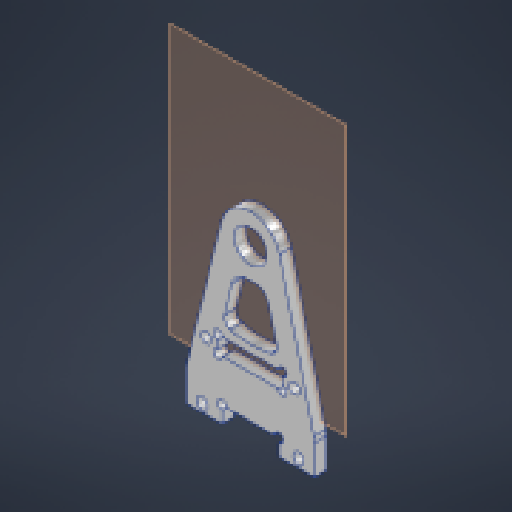
# Autodesk Inventor part: Roll_Fixation_Frame_2t1
Saved by Autodesk Inventor 2024 (Build 280153000, 153)
## iProperties
Created: 2024-01-23
Part Number: Roll_Fixation_Frame_2t1
Material: 알루미늄 6061
Document SubType Name: Modeling
Designer: ASUS
Density: 2.7 g/cm^3
Appearance: 알루미늄 - 평지
Author: ASUS
Autodesk Inventor part; units mm, degrees
(part 1 of 3)
ref_plane "YZ Plane" through (0, 0, 0) normal (1, 0, 0) x (0, 1, 0)
ref_plane "XZ Plane" through (0, 0, 0) normal (0, 1, 0) x (-1, 0, 0)
ref_plane "XY Plane" through (0, 0, 0) normal (0, 0, 1) x (1, 0, 0)
ref_plane "작업 평면1" through (0, 0, 0) normal (0, 0, 1) x (1, 0, 0)
sketch "스케치1" plane through (0, 0, 0) normal (0, 0, 1) x (1, 0, 0)
  circle A0 centre (0.1, -20) radius 6 projected
  circle A1 centre (0.1, -20) radius 4 projected
  line L0 (-13.4121, -48.1) -> (13.4121, -48.1) projected
  line L1 (0.1, -20) -> (0.1, -60)
  line L2 (0.1, -60) -> (-15.9, -60)
  line L3 (-15.9, -60) -> (-5.7269, -18.5692)
  line L4 (0.1, -60) -> (16.1, -60)
  line L5 (16.1, -60) -> (5.9269, -18.5692)
  line L6 (0.1, -48.1) -> (0.1, -60)
  line L7 (7.6, -52.05) -> (-7.4, -52.05)
  line L8 (-7.4, -52.05) -> (-7.4, -56.05)
  line L9 (-7.4, -56.05) -> (7.6, -56.05)
  line L10 (7.6, -56.05) -> (7.6, -52.05)
  line L11 (7.6, -52.05) -> (-7.4, -56.05) construction
  line L12 (-7.4, -52.05) -> (7.6, -56.05) construction
  line L13 (-7.4, -54.05) -> (-10.4, -54.05)
  line L14 (7.6, -54.05) -> (10.6, -54.05)
  circle A2 centre (10.6, -54.05) radius 1.35
  circle A3 centre (-10.4, -54.05) radius 1.35
  line L15 (7.6, -56.05) -> (7.6, -52.05) construction
  line L16 (-34.247, -53.3276) -> (-34.247, -49.3276)
  line L17 (-37.747, -49.3276) -> (-37.747, -53.3276)
  arc A4 (-37.747, -53.3276) -> (-34.247, -53.3276) centre (-35.997, -53.3276) ccw
  arc A5 (-34.247, -49.3276) -> (-37.747, -49.3276) centre (-35.997, -49.3276) ccw
  line L18 (4.1, -52.05) -> (4.1, -56.05)
  line L19 (7.6, -56.05) -> (7.6, -52.05)
  arc A6 (7.6, -52.05) -> (4.1, -52.05) centre (5.85, -52.05) ccw
  arc A7 (4.1, -56.05) -> (7.6, -56.05) centre (5.85, -56.05) ccw
  line L20 (-7.4, -52.05) -> (-7.4, -56.05)
  line L21 (-3.9, -56.05) -> (-3.9, -52.05)
  arc A8 (-3.9, -52.05) -> (-7.4, -52.05) centre (-5.65, -52.05) ccw
  arc A9 (-7.4, -56.05) -> (-3.9, -56.05) centre (-5.65, -56.05) ccw
  line L22 (-10.4, -54.05) -> (-22.3103, -54.05)
  line L23 (-22.3103, -54.05) -> (17.7315, -54.05)
  line L24 (14.639, -54.05) -> (-14.439, -54.05)
  line L25 (-14.439, -54.05) -> (-14.439, -60)
  line L26 (-14.439, -60) -> (14.639, -60)
  line L27 (14.639, -60) -> (14.639, -54.05)
  point P0 (0, 0)
  point P1 (0.1, -54.05)
  point P2 (-32.997, -51.3276)
  point P3 (-2.65, -54.05)
  point P4 (7.6, -56.05)
  point P5 (4.1, -56.05)
  point P6 (-7.4, -52.05)
  point P7 (5.9269, -18.5692)
  dimension "d0" = 40
  dimension "d1" = 16
  dimension "d2" = 15
  dimension "d3" = 4
  dimension "d4" = 3
  dimension "d5" = 3
  dimension "d7" = 2.7
  constraints: 56 end point, 12 point on circle, 12 tangent, 8 centre point, 7 parallel, 7 point on line, 6 midpoint, 5 horizontal, 4 perpendicular, 2 coincident, 2 symmetric about line, 1 vertical, 3 other
  measures "d0" distance of L1.start L1.end
  measures "d1" distance of L1.end L2.end
  measures "d2" distance of L9.end L8.end
  measures "d3" distance of L8.end L7.end
  measures "d4" distance of L13.start L13.end
  measures "d5" distance of L14.start L14.end
  measures "d7" diameter of A3
extrude "돌출1" add sketch "스케치1" along normal blind 3 contours A0 | A0 L5 L0 L1 | L1 L0 L3 A0 | L5 L23 A2 L14 L10 A6 L7 L1 L0 | L1 L7 A8 L8 L13 A3 L22 L3 L0 | L27 L4 L1 L9 A7 L10 L14 A2 L23 | L22 A3 L13 L8 A9 L9 L1 L2 L25
fillet "모깎기1" radius 4 2 edges at (14.639, -60, 1.5) (-14.439, -60, 1.5)
sketch "스케치2" plane through (0, 0, 3) normal (0, 0, 1) x (1, 0, 0)
  arc A0 (-14.439, -56) -> (-10.439, -60) centre (-10.439, -56) ccw projected
  line L0 (-10.439, -60) -> (10.639, -60) projected
  arc A1 (10.639, -60) -> (14.639, -56) centre (10.639, -56) ccw projected
  line L1 (14.639, -56) -> (14.639, -54.05) projected
  line L2 (14.639, -54.05) -> (5.9269, -18.5692) projected
  arc A2 (5.9269, -18.5692) -> (-5.7269, -18.5692) centre (0.1, -20) ccw projected
  line L3 (-5.7269, -18.5692) -> (-14.439, -54.05) projected
  line L4 (-14.439, -54.05) -> (-14.439, -56) projected
  line L5 (7.6, -52.05) -> (7.6, -56.05) projected
  arc A3 (4.1, -56.05) -> (7.6, -56.05) centre (5.85, -56.05) ccw projected
  line L6 (4.1, -56.05) -> (-3.9, -56.05) projected
  arc A4 (-7.4, -56.05) -> (-3.9, -56.05) centre (-5.65, -56.05) ccw projected
  line L7 (-7.4, -56.05) -> (-7.4, -52.05) projected
  arc A5 (-3.9, -52.05) -> (-7.4, -52.05) centre (-5.65, -52.05) ccw projected
  line L8 (-3.9, -52.05) -> (4.1, -52.05) projected
  arc A6 (7.6, -52.05) -> (4.1, -52.05) centre (5.85, -52.05) ccw projected
  circle A7 centre (10.6, -54.05) radius 1.35 projected
  circle A8 centre (0.1, -20) radius 4 projected
  circle A9 centre (-10.4, -54.05) radius 1.35 projected
  line L9 (-10.439, -54.5339) -> (-1.8423, -19.5231)
  arc A10 (2.0423, -19.5231) -> (-1.8423, -19.5231) centre (0.1, -20) ccw
  line L10 (2.0423, -19.5231) -> (10.639, -54.5339)
  line L11 (10.639, -54.5339) -> (10.639, -56)
  line L12 (10.639, -56) -> (-10.439, -56)
  line L13 (-10.439, -56) -> (-10.439, -54.5339)
  circle A11 centre (0.1, -20) radius 7.5
  circle A12 centre (0.1, -20) radius 27.5
  point P0 (0, 0)
  point P1 (-8.3826, -46.159)
  point P2 (8.5826, -46.159)
  point P3 (3.766, -26.543)
  point P4 (-3.566, -26.543)
  dimension "d14" = 4
  dimension "d15" = 15
  dimension "d16" = 20
  constraints: 10 end point, 3 centre point, 2 point on circle, 1 coincident, 5 other
  measures "d14" distance between parallel lines of L3 L9
  measures "d15" diameter of A11
  measures "d16" radial gap between concentric circles of A11 A12
extrude "돌출2" cut sketch "스케치2" against normal through all contours L9 A11 L10 A12
fillet "모깎기2" radius 4 4 edges at (3.766, -26.543, 1.5) (-3.566, -26.543, 1.5) (-8.3826, -46.159, 1.5) (8.5826, -46.159, 1.5)
sketch "스케치3" plane through (0, 0, 3) normal (0, 0, 1) x (1, 0, 0)
  arc A0 (-0.3945, -27.4837) -> (0.5945, -27.4837) centre (0.1, -20) ccw projected
  arc A1 (4.7428, -30.5211) -> (0.5945, -27.4837) centre (0.8582, -31.475) ccw projected
  line L0 (4.7428, -30.5211) -> (7.6258, -42.2624) projected
  arc A2 (4.361, -47.1679) -> (7.6258, -42.2624) centre (3.7412, -43.2162) ccw projected
  arc A3 (-4.161, -47.1679) -> (4.361, -47.1679) centre (0.1, -20) ccw projected
  arc A4 (-7.4258, -42.2624) -> (-4.161, -47.1679) centre (-3.5412, -43.2162) ccw projected
  line L1 (-7.4258, -42.2624) -> (-4.5428, -30.5211) projected
  arc A5 (-0.3945, -27.4837) -> (-4.5428, -30.5211) centre (-0.6582, -31.475) ccw projected
  arc A6 (-14.439, -56) -> (-10.439, -60) centre (-10.439, -56) ccw projected
  line L2 (-10.439, -60) -> (10.639, -60) projected
  arc A7 (10.639, -60) -> (14.639, -56) centre (10.639, -56) ccw projected
  line L3 (14.639, -56) -> (14.639, -54.05) projected
  line L4 (14.639, -54.05) -> (5.9269, -18.5692) projected
  arc A8 (5.9269, -18.5692) -> (-5.7269, -18.5692) centre (0.1, -20) ccw projected
  line L5 (-5.7269, -18.5692) -> (-14.439, -54.05) projected
  line L6 (-14.439, -54.05) -> (-14.439, -56) projected
  line L7 (7.6, -52.05) -> (7.6, -56.05) projected
  arc A9 (4.1, -56.05) -> (7.6, -56.05) centre (5.85, -56.05) ccw projected
  line L8 (4.1, -56.05) -> (-3.9, -56.05) projected
  arc A10 (-7.4, -56.05) -> (-3.9, -56.05) centre (-5.65, -56.05) ccw projected
  line L9 (-7.4, -56.05) -> (-7.4, -52.05) projected
  arc A11 (-3.9, -52.05) -> (-7.4, -52.05) centre (-5.65, -52.05) ccw projected
  line L10 (-3.9, -52.05) -> (4.1, -52.05) projected
  arc A12 (7.6, -52.05) -> (4.1, -52.05) centre (5.85, -52.05) ccw projected
  circle A13 centre (10.6, -54.05) radius 1.35 projected
  circle A14 centre (0.1, -20) radius 4 projected
  circle A15 centre (-10.4, -54.05) radius 1.35 projected
  line L11 (14.639, -54.05) -> (-14.439, -54.05)
  line L12 (-14.439, -54.05) -> (-14.439, -60)
  line L13 (-14.439, -60) -> (14.639, -60)
  line L14 (14.639, -60) -> (14.639, -54.05)
  line L15 (7.639, -58) -> (7.639, -62)
  arc A16 (4.139, -62) -> (7.639, -62) centre (5.889, -62) ccw
  line L16 (4.139, -62) -> (-3.861, -62)
  arc A17 (-7.361, -62) -> (-3.861, -62) centre (-5.611, -62) ccw
  line L17 (-7.361, -62) -> (-7.361, -58)
  arc A18 (-3.861, -58) -> (-7.361, -58) centre (-5.611, -58) ccw
  line L18 (-3.861, -58) -> (4.139, -58)
  arc A19 (7.639, -58) -> (4.139, -58) centre (5.889, -58) ccw
  circle A20 centre (10.639, -60) radius 1.35
  circle A21 centre (-10.361, -60) radius 1.35
  line L19 (10.6, -54.05) -> (10.639, -60)
  line L20 (14.639, -54.05) -> (-14.439, -54.05)
  line L21 (-14.439, -54.05) -> (-14.439, -66.05)
  line L22 (-14.439, -66.05) -> (14.639, -66.05)
  line L23 (14.639, -66.05) -> (14.639, -54.05)
  point P0 (0, 0)
  point P1 (-10.4, -61.95)
  point P2 (10.678, -61.95)
  point P3 (11.9697, -59.7722)
  point P4 (9.289, -60)
  point P5 (7.639, -60)
  point P6 (-7.361, -60)
  point P7 (-9.011, -60)
  point P8 (-11.6957, -59.7975)
  point P9 (4.4167, -57.0541)
  point P10 (7.3223, -56.9959)
  point P11 (-7.0833, -57.0541)
  point P12 (-4.1777, -56.9959)
  point P13 (11.95, -54.05)
  point P14 (10.6089, -55.4)
  dimension "d20" = 12
  constraints: 26 end point, 8 point on circle, 6 centre point, 5 equal length, 2 perpendicular, 1 horizontal
  measures "d20" distance of L21.end L5.end
extrude "돌출3" add sketch "스케치3" against normal up to surface (3 mm away) contours A6 A21 L13 L12 | L13 A21 L2 L17 A17 L16 A16 L15 A20 L23 L22 L21 | L11 A15 | A15 L11 | L11 L7 A9 A19 L8 A10 A18 L9 | L9 A11 L10 A12 L7 L11 | L13 A20 A7 L14 | L11 A13 | A13 L19 L11 | L11 L19 A13
sketch "스케치4" plane through (0, 0, 3) normal (0, 0, 1) x (1, 0, 0)
  line L0 (14.639, -66.05) -> (14.639, -54.05) projected
  line L1 (14.639, -54.05) -> (5.9269, -18.5692) projected
  arc A0 (5.9269, -18.5692) -> (-5.7269, -18.5692) centre (0.1, -20) ccw projected
  line L2 (-5.7269, -18.5692) -> (-14.439, -54.05) projected
  line L3 (-14.439, -54.05) -> (-14.439, -66.05) projected
  line L4 (-14.439, -66.05) -> (14.639, -66.05) projected
  arc A1 (9.289, -60) -> (11.9697, -59.7722) centre (10.639, -60) ccw projected
  line L5 (9.289, -60) -> (10.639, -60) projected
  arc A2 (10.639, -60) -> (11.9697, -59.7722) centre (10.639, -56) ccw projected
  line L6 (7.639, -60) -> (7.639, -62) projected
  arc A3 (4.139, -62) -> (7.639, -62) centre (5.889, -62) ccw projected
  line L7 (4.139, -62) -> (-3.861, -62) projected
  arc A4 (-7.361, -62) -> (-3.861, -62) centre (-5.611, -62) ccw projected
  line L8 (-7.361, -62) -> (-7.361, -60) projected
  line L9 (-7.361, -60) -> (7.639, -60) projected
  arc A5 (-7.0833, -57.0541) -> (-4.1777, -56.9959) centre (-5.65, -56.05) ccw projected
  arc A6 (-4.1777, -56.9959) -> (-7.0833, -57.0541) centre (-5.611, -58) ccw projected
  arc A7 (-0.3945, -27.4837) -> (0.5945, -27.4837) centre (0.1, -20) ccw projected
  arc A8 (4.7428, -30.5211) -> (0.5945, -27.4837) centre (0.8582, -31.475) ccw projected
  line L10 (4.7428, -30.5211) -> (7.6258, -42.2624) projected
  arc A9 (4.361, -47.1679) -> (7.6258, -42.2624) centre (3.7412, -43.2162) ccw projected
  arc A10 (-4.161, -47.1679) -> (4.361, -47.1679) centre (0.1, -20) ccw projected
  arc A11 (-7.4258, -42.2624) -> (-4.161, -47.1679) centre (-3.5412, -43.2162) ccw projected
  line L11 (-7.4258, -42.2624) -> (-4.5428, -30.5211) projected
  arc A12 (-0.3945, -27.4837) -> (-4.5428, -30.5211) centre (-0.6582, -31.475) ccw projected
  arc A13 (-11.6957, -59.7975) -> (-9.011, -60) centre (-10.361, -60) ccw projected
  arc A14 (-11.6957, -59.7975) -> (-10.439, -60) centre (-10.439, -56) ccw projected
  line L12 (-10.439, -60) -> (-9.011, -60) projected
  arc A15 (7.3223, -56.9959) -> (4.4167, -57.0541) centre (5.889, -58) ccw projected
  arc A16 (4.4167, -57.0541) -> (7.3223, -56.9959) centre (5.85, -56.05) ccw projected
  circle A17 centre (0.1, -20) radius 4 projected
  circle A18 centre (10.639, -60) radius 1.35
  circle A19 centre (-10.361, -60) radius 1.35
  line L13 (5.889, -58) -> (5.889, -62) construction
  line L14 (7.639, -58) -> (7.639, -62)
  line L15 (4.139, -62) -> (4.139, -58)
  arc A20 (7.639, -58) -> (4.139, -58) centre (5.889, -58) ccw
  arc A21 (4.139, -62) -> (7.639, -62) centre (5.889, -62) ccw
  line L16 (-5.611, -62) -> (-5.611, -58) construction
  line L17 (-3.861, -62) -> (-3.861, -58)
  line L18 (-7.361, -58) -> (-7.361, -62)
  arc A22 (-7.361, -62) -> (-3.861, -62) centre (-5.611, -62) ccw
  arc A23 (-3.861, -58) -> (-7.361, -58) centre (-5.611, -58) ccw
  line L19 (4.139, -58) -> (-3.861, -58)
  line L20 (-3.861, -58) -> (-3.861, -62)
  line L21 (-3.861, -62) -> (4.139, -62)
  line L22 (4.139, -62) -> (4.139, -58)
  line L23 (4.139, -58) -> (-3.861, -62) construction
  line L24 (-3.861, -58) -> (4.139, -62) construction
  point P0 (0, 0)
  point P1 (5.889, -60)
  point P2 (-5.611, -60)
  point P3 (0.139, -60)
  point P4 (-11.6957, -59.7975)
  point P5 (-4.1777, -56.9959)
  point P6 (-7.0833, -57.0541)
  point P7 (7.3223, -56.9959)
  constraints: 28 end point, 8 point on circle, 8 tangent, 5 midpoint, 5 parallel, 4 centre point, 2 coincident, 1 horizontal, 1 perpendicular, 1 vertical, 6 other
extrude "돌출4" cut sketch "스케치4" against normal through all contours A18 A2 L5 | L9 L15 A20 A16 L14 | L9 L17 L19 L15 | L9 L18 A23 A5 L17 | A19 L12 A14
sketch "스케치5" plane through (0, 0, 3) normal (0, 0, 1) x (1, 0, 0)
  circle A0 centre (10.639, -60) radius 1.35 projected
  line L0 (14.639, -66.05) -> (14.639, -54.05) projected
  line L1 (14.639, -54.05) -> (5.9269, -18.5692) projected
  arc A1 (5.9269, -18.5692) -> (-5.7269, -18.5692) centre (0.1, -20) ccw projected
  line L2 (-5.7269, -18.5692) -> (-14.439, -54.05) projected
  line L3 (-14.439, -54.05) -> (-14.439, -66.05) projected
  line L4 (-14.439, -66.05) -> (14.639, -66.05) projected
  arc A2 (-0.3945, -27.4837) -> (0.5945, -27.4837) centre (0.1, -20) ccw projected
  arc A3 (4.7428, -30.5211) -> (0.5945, -27.4837) centre (0.8582, -31.475) ccw projected
  line L5 (4.7428, -30.5211) -> (7.6258, -42.2624) projected
  arc A4 (4.361, -47.1679) -> (7.6258, -42.2624) centre (3.7412, -43.2162) ccw projected
  arc A5 (-4.161, -47.1679) -> (4.361, -47.1679) centre (0.1, -20) ccw projected
  arc A6 (-7.4258, -42.2624) -> (-4.161, -47.1679) centre (-3.5412, -43.2162) ccw projected
  line L6 (-7.4258, -42.2624) -> (-4.5428, -30.5211) projected
  arc A7 (-0.3945, -27.4837) -> (-4.5428, -30.5211) centre (-0.6582, -31.475) ccw projected
  circle A8 centre (-10.361, -60) radius 1.35 projected
  line L7 (-7.361, -62) -> (-7.361, -58) projected
  arc A9 (-3.861, -58) -> (-7.361, -58) centre (-5.611, -58) ccw projected
  line L8 (-3.861, -58) -> (4.139, -58) projected
  arc A10 (7.639, -58) -> (4.139, -58) centre (5.889, -58) ccw projected
  line L9 (7.639, -58) -> (7.639, -62) projected
  arc A11 (4.139, -62) -> (7.639, -62) centre (5.889, -62) ccw projected
  line L10 (4.139, -62) -> (-3.861, -62) projected
  arc A12 (-7.361, -62) -> (-3.861, -62) centre (-5.611, -62) ccw projected
  circle A13 centre (0.1, -20) radius 4 projected
  circle A14 centre (0.1, -20) radius 7.5
  circle A15 centre (0.1, -20) radius 32.5
  line L11 (7.6258, -42.2624) -> (10.5269, -54.0775)
  line L12 (-7.4258, -42.2624) -> (-10.5544, -55.0038)
  line L13 (4.7428, -30.5211) -> (3.4771, -25.3664)
  arc A16 (-0.3945, -27.4837) -> (-4.5428, -30.5211) centre (-0.6582, -31.475) ccw projected
  line L14 (-4.5428, -30.5211) -> (-2.9181, -23.9045)
  line L15 (-7.4258, -42.2624) -> (-4.5428, -30.5211) projected
  line L16 (4.7428, -30.5211) -> (7.6258, -42.2624) projected
  point P0 (0, 0)
  point P1 (-3.566, -26.543)
  point P2 (-0.3945, -27.4837)
  point P3 (3.766, -26.543)
  point P4 (0.5945, -27.4837)
  point P5 (-9.5776, -51.0257)
  point P6 (9.7776, -51.0257)
  dimension "d25" = 65
  constraints: 8 end point, 3 collinear, 2 centre point, 2 coincident, 1 tangent
  measures "d25" diameter of A15
extrude "돌출5" cut sketch "스케치5" against normal through all contours A15 L12 A6 A5 A4 L11 | L13 A3 A14 | A14 A7 L14
fillet "모깎기3" radius 4 4 edges at (9.7776, -51.0257, 1.5) (-9.5776, -51.0257, 1.5) (-3.566, -26.543, 1.5) (3.766, -26.543, 1.5)
fillet "모깎기4" radius 4 4 edges at (14.639, -66.05, 1.5) (-14.439, -66.05, 1.5) (14.639, -54.05, 1.5) (-14.439, -54.05, 1.5)
sketch "스케치6" plane through (0, 0, 3) normal (0, 0, 1) x (1, 0, 0)
  circle A0 centre (10.639, -60) radius 1.35 projected
  line L0 (-8.6217, -47.1327) -> (-4.5428, -30.5211) projected
  arc A1 (-0.3945, -27.4837) -> (-4.5428, -30.5211) centre (-0.6582, -31.475) ccw projected
  arc A2 (-0.3945, -27.4837) -> (0.5945, -27.4837) centre (0.1, -20) ccw projected
  arc A3 (4.7428, -30.5211) -> (0.5945, -27.4837) centre (0.8582, -31.475) ccw projected
  line L1 (4.7428, -30.5211) -> (8.8217, -47.1327) projected
  arc A4 (5.616, -52.0285) -> (8.8217, -47.1327) centre (4.9371, -48.0865) ccw projected
  arc A5 (-5.416, -52.0285) -> (5.616, -52.0285) centre (0.1, -20) ccw projected
  arc A6 (-8.6217, -47.1327) -> (-5.416, -52.0285) centre (-4.7371, -48.0865) ccw projected
  circle A7 centre (-10.361, -60) radius 1.35 projected
  line L2 (-7.361, -62) -> (-7.361, -58) projected
  arc A8 (-3.861, -58) -> (-7.361, -58) centre (-5.611, -58) ccw projected
  line L3 (-3.861, -58) -> (4.139, -58) projected
  arc A9 (7.639, -58) -> (4.139, -58) centre (5.889, -58) ccw projected
  line L4 (7.639, -58) -> (7.639, -62) projected
  arc A10 (4.139, -62) -> (7.639, -62) centre (5.889, -62) ccw projected
  line L5 (4.139, -62) -> (-3.861, -62) projected
  arc A11 (-7.361, -62) -> (-3.861, -62) centre (-5.611, -62) ccw projected
  circle A12 centre (0.1, -20) radius 4 projected
  arc A13 (-14.3236, -53.5801) -> (-14.439, -54.5339) centre (-10.439, -54.5339) ccw projected
  line L6 (-14.439, -54.5339) -> (-14.439, -62.05) projected
  arc A14 (-14.439, -62.05) -> (-10.439, -66.05) centre (-10.439, -62.05) ccw projected
  line L7 (-10.439, -66.05) -> (10.639, -66.05) projected
  arc A15 (10.639, -66.05) -> (14.639, -62.05) centre (10.639, -62.05) ccw projected
  line L8 (14.639, -62.05) -> (14.639, -54.5339) projected
  arc A16 (14.639, -54.5339) -> (14.5236, -53.5801) centre (10.639, -54.5339) ccw projected
  line L9 (14.5236, -53.5801) -> (5.9269, -18.5692) projected
  arc A17 (5.9269, -18.5692) -> (-5.7269, -18.5692) centre (0.1, -20) ccw projected
  line L10 (-5.7269, -18.5692) -> (-14.3236, -53.5801) projected
  point P0 (0, 0)
extrude "돌출6" cut sketch "스케치6" against normal blind 1
sketch "스케치7" plane through (0, 0, 0) normal (0, 0, -1) x (-1, 0, 0)
  arc A0 (14.439, -54.5339) -> (14.3236, -53.5801) centre (10.439, -54.5339) ccw projected
  line L0 (5.7269, -18.5692) -> (14.3236, -53.5801) projected
  arc A1 (5.7269, -18.5692) -> (-5.9269, -18.5692) centre (-0.1, -20) ccw projected
  line L1 (-14.5236, -53.5801) -> (-5.9269, -18.5692) projected
  arc A2 (-14.5236, -53.5801) -> (-14.639, -54.5339) centre (-10.639, -54.5339) ccw projected
  line L2 (-14.639, -62.05) -> (-14.639, -54.5339) projected
  arc A3 (-14.639, -62.05) -> (-10.639, -66.05) centre (-10.639, -62.05) ccw projected
  line L3 (-10.639, -66.05) -> (10.439, -66.05) projected
  arc A4 (10.439, -66.05) -> (14.439, -62.05) centre (10.439, -62.05) ccw projected
  line L4 (14.439, -54.5339) -> (14.439, -62.05) projected
  circle A5 centre (-0.1, -20) radius 4 projected
  circle A6 centre (-10.639, -60) radius 1.35 projected
  arc A7 (7.361, -58) -> (3.861, -58) centre (5.611, -58) ccw projected
  line L5 (7.361, -58) -> (7.361, -62) projected
  arc A8 (3.861, -62) -> (7.361, -62) centre (5.611, -62) ccw projected
  line L6 (3.861, -62) -> (-4.139, -62) projected
  arc A9 (-7.639, -62) -> (-4.139, -62) centre (-5.889, -62) ccw projected
  line L7 (-7.639, -62) -> (-7.639, -58) projected
  arc A10 (-4.139, -58) -> (-7.639, -58) centre (-5.889, -58) ccw projected
  line L8 (-4.139, -58) -> (3.861, -58) projected
  circle A11 centre (10.361, -60) radius 1.35 projected
  line L9 (4.5428, -30.5211) -> (8.6217, -47.1327) projected
  arc A12 (5.416, -52.0285) -> (8.6217, -47.1327) centre (4.7371, -48.0865) ccw projected
  arc A13 (-5.616, -52.0285) -> (5.416, -52.0285) centre (-0.1, -20) ccw projected
  arc A14 (-8.8217, -47.1327) -> (-5.616, -52.0285) centre (-4.9371, -48.0865) ccw projected
  line L10 (-8.8217, -47.1327) -> (-4.7428, -30.5211) projected
  arc A15 (-0.5945, -27.4837) -> (-4.7428, -30.5211) centre (-0.8582, -31.475) ccw projected
  arc A16 (-0.5945, -27.4837) -> (0.3945, -27.4837) centre (-0.1, -20) ccw projected
  arc A17 (4.5428, -30.5211) -> (0.3945, -27.4837) centre (0.6582, -31.475) ccw projected
  point P0 (0, 0)
extrude "돌출7" add sketch "스케치7" against normal up to surface (2 mm away) contours L9 A12 A13 A14 L10 A15 A16 A17
sketch "스케치8" plane through (0, 0, 2) normal (0, 0, 1) x (1, 0, 0)
  line L0 (-14.439, -62.05) -> (-14.439, -54.5339) projected
  arc A0 (-14.439, -62.05) -> (-10.439, -66.05) centre (-10.439, -62.05) ccw projected
  line L1 (10.639, -66.05) -> (-10.439, -66.05) projected
  arc A1 (10.639, -66.05) -> (14.639, -62.05) centre (10.639, -62.05) ccw projected
  line L2 (14.639, -54.5339) -> (14.639, -62.05) projected
  arc A2 (14.639, -54.5339) -> (14.5236, -53.5801) centre (10.639, -54.5339) ccw projected
  line L3 (5.9269, -18.5692) -> (14.5236, -53.5801) projected
  arc A3 (5.9269, -18.5692) -> (-5.7269, -18.5692) centre (0.1, -20) ccw projected
  line L4 (-14.3236, -53.5801) -> (-5.7269, -18.5692) projected
  arc A4 (-14.3236, -53.5801) -> (-14.439, -54.5339) centre (-10.439, -54.5339) ccw projected
  circle A5 centre (10.639, -60) radius 1.35 projected
  circle A6 centre (-10.361, -60) radius 1.35 projected
  circle A7 centre (0.1, -20) radius 4 projected
  line L5 (-3.861, -62) -> (4.139, -62) projected
  arc A8 (-7.361, -62) -> (-3.861, -62) centre (-5.611, -62) ccw projected
  line L6 (-7.361, -58) -> (-7.361, -62) projected
  arc A9 (-3.861, -58) -> (-7.361, -58) centre (-5.611, -58) ccw projected
  line L7 (4.139, -58) -> (-3.861, -58) projected
  arc A10 (7.639, -58) -> (4.139, -58) centre (5.889, -58) ccw projected
  line L8 (7.639, -62) -> (7.639, -58) projected
  arc A11 (4.139, -62) -> (7.639, -62) centre (5.889, -62) ccw projected
  arc A12 (7.8692, -18.0923) -> (-7.6692, -18.0923) centre (0.1, -20) ccw
  line L9 (7.8692, -18.0923) -> (16.4659, -53.1031)
  arc A13 (16.639, -54.5339) -> (16.4659, -53.1031) centre (10.639, -54.5339) ccw
  line L10 (16.639, -54.5339) -> (16.639, -62.05)
  arc A14 (10.639, -68.05) -> (16.639, -62.05) centre (10.639, -62.05) ccw
  line L11 (10.639, -68.05) -> (-10.439, -68.05)
  arc A15 (-16.439, -62.05) -> (-10.439, -68.05) centre (-10.439, -62.05) ccw
  line L12 (-16.439, -62.05) -> (-16.439, -54.5339)
  arc A16 (-16.2659, -53.1031) -> (-16.439, -54.5339) centre (-10.439, -54.5339) ccw
  line L13 (-16.2659, -53.1031) -> (-7.6692, -18.0923)
  point P0 (0, 0)
  dimension "d34" = 2
  constraints: 10 end point, 10 point on circle, 5 centre point, 9 other
  measures "d34" distance between parallel lines of L4 L13
extrude "돌출8" add sketch "스케치8" against normal blind 2 contours L9 A13 L10 A14 L11 A15 L12 A16 L13 A12
sketch "스케치9" plane through (0, 0, 0) normal (0, 0, -1) x (-1, 0, 0)
  line L0 (-7.8692, -18.0923) -> (-16.4659, -53.1031) projected
  arc A0 (-16.4659, -53.1031) -> (-16.639, -54.5339) centre (-10.639, -54.5339) ccw projected
  line L1 (-16.639, -54.5339) -> (-16.639, -62.05) projected
  arc A1 (-16.639, -62.05) -> (-10.639, -68.05) centre (-10.639, -62.05) ccw projected
  line L2 (-10.639, -68.05) -> (10.439, -68.05) projected
  arc A2 (10.439, -68.05) -> (16.439, -62.05) centre (10.439, -62.05) ccw projected
  line L3 (16.439, -62.05) -> (16.439, -54.5339) projected
  arc A3 (16.439, -54.5339) -> (16.2659, -53.1031) centre (10.439, -54.5339) ccw projected
  line L4 (16.2659, -53.1031) -> (7.6692, -18.0923) projected
  arc A4 (7.6692, -18.0923) -> (-7.8692, -18.0923) centre (-0.1, -20) ccw projected
  circle A5 centre (-0.1, -20) radius 4 projected
  circle A6 centre (-10.639, -60) radius 1.35 projected
  arc A7 (7.361, -58) -> (3.861, -58) centre (5.611, -58) ccw projected
  line L5 (7.361, -58) -> (7.361, -62) projected
  arc A8 (3.861, -62) -> (7.361, -62) centre (5.611, -62) ccw projected
  line L6 (3.861, -62) -> (-4.139, -62) projected
  arc A9 (-7.639, -62) -> (-4.139, -62) centre (-5.889, -62) ccw projected
  line L7 (-7.639, -62) -> (-7.639, -58) projected
  arc A10 (-4.139, -58) -> (-7.639, -58) centre (-5.889, -58) ccw projected
  line L8 (-4.139, -58) -> (3.861, -58) projected
  circle A11 centre (10.361, -60) radius 1.35 projected
  arc A12 (-19.6808, 6.2636) -> (-20.2, 4.5766) centre (-17.2, 4.5766) ccw projected
  line L9 (-19.6808, 6.2636) -> (-15.6953, 12.1246) projected
  arc A13 (-14.0414, 13) -> (-15.6953, 12.1246) centre (-14.0414, 11) ccw projected
  line L10 (-13.1, 13) -> (-14.0414, 13) projected
  arc A14 (-13.1, 13) -> (-14.6, 11.5) centre (-13.1, 11.5) ccw projected
  line L11 (-14.6, -41.5) -> (-14.6, 11.5) projected
  arc A15 (-14.6, -41.5) -> (-13.6, -42.5) centre (-13.6, -41.5) ccw projected
  line L12 (13.4, -42.5) -> (-13.6, -42.5) projected
  arc A16 (13.4, -42.5) -> (14.4, -41.5) centre (13.4, -41.5) ccw projected
  line L13 (14.4, 11.5) -> (14.4, -41.5) projected
  arc A17 (14.4, 11.5) -> (12.9, 13) centre (12.9, 11.5) ccw projected
  line L14 (13.8414, 13) -> (12.9, 13) projected
  arc A18 (15.4953, 12.1246) -> (13.8414, 13) centre (13.8414, 11) ccw projected
  line L15 (15.4953, 12.1246) -> (19.4808, 6.2636) projected
  arc A19 (20, 4.5766) -> (19.4808, 6.2636) centre (17, 4.5766) ccw projected
  line L16 (20, 4.5766) -> (20, -39.6766) projected
  arc A20 (19.4808, -41.3636) -> (20, -39.6766) centre (17, -39.6766) ccw projected
  line L17 (19.4808, -41.3636) -> (15.7929, -46.7869) projected
  arc A21 (13.3121, -48.1) -> (15.7929, -46.7869) centre (13.3121, -45.1) ccw projected
  line L18 (13.3121, -48.1) -> (-13.5121, -48.1) projected
  arc A22 (-15.9929, -46.7869) -> (-13.5121, -48.1) centre (-13.5121, -45.1) ccw projected
  line L19 (-15.9929, -46.7869) -> (-19.6808, -41.3636) projected
  arc A23 (-20.2, -39.6766) -> (-19.6808, -41.3636) centre (-17.2, -39.6766) ccw projected
  line L20 (-20.2, -39.6766) -> (-20.2, 4.5766) projected
  circle A24 centre (17.2, 4) radius 1.35 projected
  circle A25 centre (17.2, -18) radius 1.35 projected
  circle A26 centre (10.9, -45.3) radius 1.35 projected
  circle A27 centre (-17.4, 4) radius 1.35 projected
  circle A28 centre (-17.4, -18) radius 1.35 projected
  circle A29 centre (-11.1, -45.3) radius 1.35 projected
  circle A30 centre (17.2, -40) radius 1.35 projected
  circle A31 centre (-17.4, -40) radius 1.35 projected
  line L21 (10.9, -45.3) -> (-11.1, -45.3)
  line L22 (-6.1, -43.3) -> (5.9, -43.3)
  line L23 (5.9, -43.3) -> (5.9, -47.3)
  line L24 (5.9, -47.3) -> (-6.1, -47.3)
  line L25 (-6.1, -47.3) -> (-6.1, -43.3)
  line L26 (-6.1, -43.3) -> (5.9, -47.3) construction
  line L27 (5.9, -43.3) -> (-6.1, -47.3) construction
  line L28 (5.9, -47.3) -> (5.9, -43.3) construction
  line L29 (7.9, -47.3) -> (7.9, -43.3)
  line L30 (3.9, -43.3) -> (3.9, -47.3)
  arc A32 (3.9, -47.3) -> (7.9, -47.3) centre (5.9, -47.3) ccw
  arc A33 (7.9, -43.3) -> (3.9, -43.3) centre (5.9, -43.3) ccw
  line L31 (-6.1, -47.3) -> (-6.1, -43.3) construction
  line L32 (-4.1, -47.3) -> (-4.1, -43.3)
  line L33 (-8.1, -43.3) -> (-8.1, -47.3)
  arc A34 (-8.1, -47.3) -> (-4.1, -47.3) centre (-6.1, -47.3) ccw
  arc A35 (-4.1, -43.3) -> (-8.1, -43.3) centre (-6.1, -43.3) ccw
  point P0 (0, 0)
  point P1 (-0.1, -45.3)
  point P2 (5.9, -45.3)
  point P3 (-6.1, -45.3)
  point P4 (3.9, -47.3)
  point P5 (-4.1, -43.3)
  dimension "d37" = 12
  dimension "d38" = 4
  dimension "d39" = 4
  dimension "d40" = 4
  constraints: 30 end point, 8 point on circle, 8 tangent, 5 midpoint, 4 centre point, 4 parallel, 3 perpendicular, 2 horizontal
  measures "d37" distance of L23.end L24.end
  measures "d38" distance of L22.end L23.end
  measures "d39" diameter of A33
  measures "d40" diameter of A35
extrude "돌출9" cut sketch "스케치9" against normal through all contours A35 L12 | L12 A35 L22 L25 L21 L33 | A34 L33 L21 L25 L24 L18 | L18 A34 | A33 L29 L21 L23 L22 L12 | L12 A33 | L32 L21 L25 L22 | L22 L30 L21 L32 | A32 L18 | L18 A32 L24 L23 L21 L29 | L32 L21 L30 L24 | L24 L25 L21 L32 | L22 L23 L21 L30 | L30 L21 L23 L24 | A26 | A29
sketch "스케치10" plane through (0, 0, 0) normal (0, 0, -1) x (-1, 0, 0)
  circle A0 centre (-11.1, -45.3) radius 1.35 projected
  circle A1 centre (10.9, -45.3) radius 1.35 projected
  arc A2 (7.9, -43.3) -> (3.9, -43.3) centre (5.9, -43.3) ccw projected
  line L0 (7.9, -43.3) -> (7.9, -47.3) projected
  arc A3 (3.9, -47.3) -> (7.9, -47.3) centre (5.9, -47.3) ccw projected
  line L1 (3.9, -47.3) -> (-4.1, -47.3) projected
  arc A4 (-8.1, -47.3) -> (-4.1, -47.3) centre (-6.1, -47.3) ccw projected
  line L2 (-8.1, -47.3) -> (-8.1, -43.3) projected
  arc A5 (-4.1, -43.3) -> (-8.1, -43.3) centre (-6.1, -43.3) ccw projected
  line L3 (-4.1, -43.3) -> (3.9, -43.3) projected
  line L4 (-7.8692, -18.0923) -> (-16.4659, -53.1031) projected
  arc A6 (-16.4659, -53.1031) -> (-16.639, -54.5339) centre (-10.639, -54.5339) ccw projected
  line L5 (-16.639, -54.5339) -> (-16.639, -62.05) projected
  arc A7 (-16.639, -62.05) -> (-10.639, -68.05) centre (-10.639, -62.05) ccw projected
  line L6 (-10.639, -68.05) -> (10.439, -68.05) projected
  arc A8 (10.439, -68.05) -> (16.439, -62.05) centre (10.439, -62.05) ccw projected
  line L7 (16.439, -62.05) -> (16.439, -54.5339) projected
  arc A9 (16.439, -54.5339) -> (16.2659, -53.1031) centre (10.439, -54.5339) ccw projected
  line L8 (16.2659, -53.1031) -> (7.6692, -18.0923) projected
  arc A10 (7.6692, -18.0923) -> (-7.8692, -18.0923) centre (-0.1, -20) ccw projected
  circle A11 centre (-0.1, -20) radius 4 projected
  circle A12 centre (-10.639, -60) radius 1.35 projected
  arc A13 (7.361, -58) -> (3.861, -58) centre (5.611, -58) ccw projected
  line L9 (7.361, -58) -> (7.361, -62) projected
  arc A14 (3.861, -62) -> (7.361, -62) centre (5.611, -62) ccw projected
  line L10 (3.861, -62) -> (-4.139, -62) projected
  arc A15 (-7.639, -62) -> (-4.139, -62) centre (-5.889, -62) ccw projected
  line L11 (-7.639, -62) -> (-7.639, -58) projected
  arc A16 (-4.139, -58) -> (-7.639, -58) centre (-5.889, -58) ccw projected
  line L12 (-4.139, -58) -> (3.861, -58) projected
  circle A17 centre (10.361, -60) radius 1.35 projected
  circle A18 centre (-0.1, -20) radius 8
  line L13 (-0.139, -62) -> (-0.1, -43.3)
  circle A19 centre (-0.1, -20) radius 20
  line L14 (2.8135, -19.2846) -> (11.4102, -54.2954)
  arc A20 (11.439, -54.5339) -> (11.4102, -54.2954) centre (10.439, -54.5339) ccw
  line L15 (11.439, -54.5339) -> (11.439, -62.05)
  arc A21 (10.439, -63.05) -> (11.439, -62.05) centre (10.439, -62.05) ccw
  line L16 (10.439, -63.05) -> (-10.639, -63.05)
  arc A22 (-11.639, -62.05) -> (-10.639, -63.05) centre (-10.639, -62.05) ccw
  line L17 (-11.639, -62.05) -> (-11.639, -54.5339)
  arc A23 (-11.6102, -54.2954) -> (-11.639, -54.5339) centre (-10.639, -54.5339) ccw
  line L18 (-11.6102, -54.2954) -> (-3.0135, -19.2846)
  arc A24 (2.8135, -19.2846) -> (-3.0135, -19.2846) centre (-0.1, -20) ccw
  point P0 (0, 0)
  point P1 (-4.7819, -26.4869)
  point P2 (-7.7287, -38.4879)
  point P3 (7.5287, -38.4879)
  point P4 (4.5819, -26.4869)
  dimension "d43" = 40
  dimension "d44" = 5
  constraints: 12 end point, 10 point on circle, 7 centre point, 2 coincident, 2 midpoint, 1 concentric, 9 other
  measures "d43" diameter of A19
  measures "d44" distance between parallel lines of L8 L14
extrude "돌출10" cut sketch "스케치10" against normal through all contours A18 L14 A19 L18
fillet "모깎기5" radius 2 4 edges at (-7.5287, -38.4879, 1) (-4.5819, -26.4869, 1) (4.7819, -26.4869, 1) (7.7287, -38.4879, 1)
sketch "스케치11" plane through (0, 0, 2) normal (0, 0, 1) x (1, 0, 0)
  line L0 (-7.0991, -36.7384) -> (-5.1861, -28.9475) projected
  arc A0 (-2.575, -27.5395) -> (-5.1861, -28.9475) centre (-3.2438, -29.4244) ccw projected
  arc A1 (-2.575, -27.5395) -> (2.775, -27.5395) centre (0.1, -20) ccw projected
  arc A2 (5.3861, -28.9475) -> (2.775, -27.5395) centre (3.4438, -29.4244) ccw projected
  line L1 (5.3861, -28.9475) -> (7.2991, -36.7384) projected
  arc A3 (5.9409, -39.1281) -> (7.2991, -36.7384) centre (5.3568, -37.2153) ccw projected
  arc A4 (-5.7409, -39.1281) -> (5.9409, -39.1281) centre (0.1, -20) ccw projected
  arc A5 (-7.0991, -36.7384) -> (-5.7409, -39.1281) centre (-5.1568, -37.2153) ccw projected
  circle A6 centre (11.1, -45.3) radius 1.35 projected
  circle A7 centre (-10.9, -45.3) radius 1.35 projected
  arc A8 (-3.9, -43.3) -> (-7.9, -43.3) centre (-5.9, -43.3) ccw projected
  line L2 (-3.9, -43.3) -> (4.1, -43.3) projected
  arc A9 (8.1, -43.3) -> (4.1, -43.3) centre (6.1, -43.3) ccw projected
  line L3 (8.1, -43.3) -> (8.1, -47.3) projected
  arc A10 (4.1, -47.3) -> (8.1, -47.3) centre (6.1, -47.3) ccw projected
  line L4 (4.1, -47.3) -> (-3.9, -47.3) projected
  arc A11 (-7.9, -47.3) -> (-3.9, -47.3) centre (-5.9, -47.3) ccw projected
  line L5 (-7.9, -47.3) -> (-7.9, -43.3) projected
  line L6 (16.4659, -53.1031) -> (7.8692, -18.0923) projected
  arc A12 (7.8692, -18.0923) -> (-7.6692, -18.0923) centre (0.1, -20) ccw projected
  line L7 (-7.6692, -18.0923) -> (-16.2659, -53.1031) projected
  arc A13 (-16.2659, -53.1031) -> (-16.439, -54.5339) centre (-10.439, -54.5339) ccw projected
  line L8 (-16.439, -54.5339) -> (-16.439, -62.05) projected
  arc A14 (-16.439, -62.05) -> (-10.439, -68.05) centre (-10.439, -62.05) ccw projected
  line L9 (-10.439, -68.05) -> (10.639, -68.05) projected
  arc A15 (10.639, -68.05) -> (16.639, -62.05) centre (10.639, -62.05) ccw projected
  line L10 (16.639, -62.05) -> (16.639, -54.5339) projected
  arc A16 (16.639, -54.5339) -> (16.4659, -53.1031) centre (10.639, -54.5339) ccw projected
  circle A17 centre (10.639, -60) radius 1.35 projected
  circle A18 centre (-10.361, -60) radius 1.35 projected
  circle A19 centre (0.1, -20) radius 4 projected
  line L11 (-3.861, -62) -> (4.139, -62) projected
  arc A20 (-7.361, -62) -> (-3.861, -62) centre (-5.611, -62) ccw projected
  line L12 (-7.361, -58) -> (-7.361, -62) projected
  arc A21 (-3.861, -58) -> (-7.361, -58) centre (-5.611, -58) ccw projected
  line L13 (4.139, -58) -> (-3.861, -58) projected
  arc A22 (7.639, -58) -> (4.139, -58) centre (5.889, -58) ccw projected
  line L14 (7.639, -62) -> (7.639, -58) projected
  arc A23 (4.139, -62) -> (7.639, -62) centre (5.889, -62) ccw projected
  line L15 (4.08, -62.06) -> (-3.802, -62.06)
  arc A24 (-7.421, -62) -> (-3.802, -62.06) centre (-5.611, -62) ccw
  line L16 (-7.421, -62) -> (-7.421, -58)
  arc A25 (-3.802, -57.94) -> (-7.421, -58) centre (-5.611, -58) ccw
  line L17 (-3.802, -57.94) -> (4.08, -57.94)
  arc A26 (7.699, -58) -> (4.08, -57.94) centre (5.889, -58) ccw
  line L18 (7.699, -58) -> (7.699, -62)
  arc A27 (4.08, -62.06) -> (7.699, -62) centre (5.889, -62) ccw
  line L19 (-3.8409, -47.36) -> (4.0409, -47.36)
  arc A28 (4.0409, -47.36) -> (8.16, -47.3) centre (6.1, -47.3) ccw
  line L20 (8.16, -47.3) -> (8.16, -43.3)
  arc A29 (8.16, -43.3) -> (4.0409, -43.24) centre (6.1, -43.3) ccw
  line L21 (4.0409, -43.24) -> (-3.8409, -43.24)
  arc A30 (-3.8409, -43.24) -> (-7.96, -43.3) centre (-5.9, -43.3) ccw
  line L22 (-7.96, -43.3) -> (-7.96, -47.3)
  arc A31 (-7.96, -47.3) -> (-3.8409, -47.36) centre (-5.9, -47.3) ccw
  point P0 (0, 0)
  dimension "d48" = 0.06
  dimension "d49" = 0.06
  constraints: 16 end point, 16 point on circle, 8 centre point, 14 other
  measures "d48" distance between parallel lines of L11 L15
  measures "d49" distance between parallel lines of L4 L19
extrude "돌출11" cut sketch "스케치11" against normal through all contours L2 A9 L3 A10 L4 A11 L5 A8 | A20 L12 A21 L13 A22 L14 A23 L11 | L15 A24 L16 A25 L17 A26 L18 A27 | A31 L22 A30 L21 A29 L20 A28 L19
sketch "스케치12" plane through (0, 0, 2) normal (0, 0, 1) x (1, 0, 0)
  line L0 (8.16, -43.3) -> (8.16, -47.3) projected
  arc A0 (4.0409, -47.36) -> (8.16, -47.3) centre (6.1, -47.3) ccw projected
  line L1 (4.0409, -47.36) -> (-3.8409, -47.36) projected
  arc A1 (-7.96, -47.3) -> (-3.8409, -47.36) centre (-5.9, -47.3) ccw projected
  line L2 (-7.96, -47.3) -> (-7.96, -43.3) projected
  arc A2 (-3.8409, -43.24) -> (-7.96, -43.3) centre (-5.9, -43.3) ccw projected
  line L3 (-3.8409, -43.24) -> (4.0409, -43.24) projected
  arc A3 (8.16, -43.3) -> (4.0409, -43.24) centre (6.1, -43.3) ccw projected
  arc A4 (-3.802, -57.94) -> (-7.421, -58) centre (-5.611, -58) ccw projected
  line L4 (-3.802, -57.94) -> (4.08, -57.94) projected
  arc A5 (7.699, -58) -> (4.08, -57.94) centre (5.889, -58) ccw projected
  line L5 (7.699, -58) -> (7.699, -62) projected
  arc A6 (4.08, -62.06) -> (7.699, -62) centre (5.889, -62) ccw projected
  line L6 (4.08, -62.06) -> (-3.802, -62.06) projected
  arc A7 (-7.421, -62) -> (-3.802, -62.06) centre (-5.611, -62) ccw projected
  line L7 (-7.421, -62) -> (-7.421, -58) projected
  line L8 (-7.0991, -36.7384) -> (-5.1861, -28.9475) projected
  arc A8 (-2.575, -27.5395) -> (-5.1861, -28.9475) centre (-3.2438, -29.4244) ccw projected
  arc A9 (-2.575, -27.5395) -> (2.775, -27.5395) centre (0.1, -20) ccw projected
  arc A10 (5.3861, -28.9475) -> (2.775, -27.5395) centre (3.4438, -29.4244) ccw projected
  line L9 (5.3861, -28.9475) -> (7.2991, -36.7384) projected
  arc A11 (5.9409, -39.1281) -> (7.2991, -36.7384) centre (5.3568, -37.2153) ccw projected
  arc A12 (-5.7409, -39.1281) -> (5.9409, -39.1281) centre (0.1, -20) ccw projected
  arc A13 (-7.0991, -36.7384) -> (-5.7409, -39.1281) centre (-5.1568, -37.2153) ccw projected
  circle A14 centre (11.1, -45.3) radius 1.35 projected
  circle A15 centre (-10.9, -45.3) radius 1.35 projected
  line L10 (16.4659, -53.1031) -> (7.8692, -18.0923) projected
  arc A16 (7.8692, -18.0923) -> (-7.6692, -18.0923) centre (0.1, -20) ccw projected
  line L11 (-7.6692, -18.0923) -> (-16.2659, -53.1031) projected
  arc A17 (-16.2659, -53.1031) -> (-16.439, -54.5339) centre (-10.439, -54.5339) ccw projected
  line L12 (-16.439, -54.5339) -> (-16.439, -62.05) projected
  arc A18 (-16.439, -62.05) -> (-10.439, -68.05) centre (-10.439, -62.05) ccw projected
  line L13 (-10.439, -68.05) -> (10.639, -68.05) projected
  arc A19 (10.639, -68.05) -> (16.639, -62.05) centre (10.639, -62.05) ccw projected
  line L14 (16.639, -62.05) -> (16.639, -54.5339) projected
  arc A20 (16.639, -54.5339) -> (16.4659, -53.1031) centre (10.639, -54.5339) ccw projected
  circle A21 centre (10.639, -60) radius 1.35 projected
  circle A22 centre (-10.361, -60) radius 1.35 projected
  circle A23 centre (0.1, -20) radius 4 projected
  circle A24 centre (10.739, -60) radius 1.35 projected
  line L15 (-8.5217, -47.1327) -> (-4.4428, -30.5211) projected
  arc A25 (-0.2945, -27.4837) -> (-4.4428, -30.5211) centre (-0.5582, -31.475) ccw projected
  arc A26 (-0.2945, -27.4837) -> (0.6945, -27.4837) centre (0.2, -20) ccw projected
  arc A27 (4.8428, -30.5211) -> (0.6945, -27.4837) centre (0.9582, -31.475) ccw projected
  line L16 (4.8428, -30.5211) -> (8.9217, -47.1327) projected
  arc A28 (5.716, -52.0285) -> (8.9217, -47.1327) centre (5.0371, -48.0865) ccw projected
  arc A29 (-5.316, -52.0285) -> (5.716, -52.0285) centre (0.2, -20) ccw projected
  arc A30 (-8.5217, -47.1327) -> (-5.316, -52.0285) centre (-4.6371, -48.0865) ccw projected
  circle A31 centre (-10.261, -60) radius 1.35 projected
  line L17 (-7.261, -62) -> (-7.261, -58) projected
  arc A32 (-3.761, -58) -> (-7.261, -58) centre (-5.511, -58) ccw projected
  line L18 (-3.761, -58) -> (4.239, -58) projected
  arc A33 (7.739, -58) -> (4.239, -58) centre (5.989, -58) ccw projected
  line L19 (7.739, -58) -> (7.739, -62) projected
  arc A34 (4.239, -62) -> (7.739, -62) centre (5.989, -62) ccw projected
  line L20 (4.239, -62) -> (-3.761, -62) projected
  arc A35 (-7.261, -62) -> (-3.761, -62) centre (-5.511, -62) ccw projected
  circle A36 centre (0.2, -20) radius 4 projected
  arc A37 (-14.2236, -53.5801) -> (-14.339, -54.5339) centre (-10.339, -54.5339) ccw projected
  line L21 (-14.339, -54.5339) -> (-14.339, -62.05) projected
  arc A38 (-14.339, -62.05) -> (-10.339, -66.05) centre (-10.339, -62.05) ccw projected
  line L22 (-10.339, -66.05) -> (10.739, -66.05) projected
  arc A39 (10.739, -66.05) -> (14.739, -62.05) centre (10.739, -62.05) ccw projected
  line L23 (14.739, -62.05) -> (14.739, -54.5339) projected
  arc A40 (14.739, -54.5339) -> (14.6236, -53.5801) centre (10.739, -54.5339) ccw projected
  line L24 (14.6236, -53.5801) -> (6.0269, -18.5692) projected
  arc A41 (6.0269, -18.5692) -> (-5.6269, -18.5692) centre (0.2, -20) ccw projected
  line L25 (-5.6269, -18.5692) -> (-14.2236, -53.5801) projected
  line L26 (10.739, -66.05) -> (16.639, -66.05)
  line L27 (16.639, -66.05) -> (16.639, -62.05)
  line L28 (16.639, -62.05) -> (10.739, -62.05)
  line L29 (10.739, -62.05) -> (10.739, -66.05)
  line L30 (-10.339, -66.05) -> (-16.439, -66.05)
  line L31 (-16.439, -66.05) -> (-16.439, -62.05)
  line L32 (-16.439, -62.05) -> (-10.339, -62.05)
  line L33 (-10.339, -62.05) -> (-10.339, -66.05)
  point P0 (0, 0)
  point P1 (15.1111, -66.05)
  point P2 (-14.9111, -66.05)
  constraints: 16 end point, 4 parallel, 2 horizontal, 2 perpendicular
extrude "돌출12" cut sketch "스케치12" against normal blind 10 contours L22 L26 A19 L13 A18 L30
sketch "스케치13" plane through (0, 0, 2) normal (0, 0, 1) x (1, 0, 0)
  circle A0 centre (0.1, -20) radius 4 projected
  circle A1 centre (-10.361, -60) radius 1.35 projected
  circle A2 centre (10.639, -60) radius 1.35 projected
  line L0 (-14.9111, -66.05) -> (15.1111, -66.05) projected
  arc A3 (15.1111, -66.05) -> (16.639, -62.05) centre (10.639, -62.05) ccw projected
  line L1 (16.639, -62.05) -> (16.639, -54.5339) projected
  arc A4 (16.639, -54.5339) -> (16.4659, -53.1031) centre (10.639, -54.5339) ccw projected
  line L2 (16.4659, -53.1031) -> (7.8692, -18.0923) projected
  arc A5 (7.8692, -18.0923) -> (-7.6692, -18.0923) centre (0.1, -20) ccw projected
  line L3 (-7.6692, -18.0923) -> (-16.2659, -53.1031) projected
  arc A6 (-16.2659, -53.1031) -> (-16.439, -54.5339) centre (-10.439, -54.5339) ccw projected
  line L4 (-16.439, -54.5339) -> (-16.439, -62.05) projected
  arc A7 (-16.439, -62.05) -> (-14.9111, -66.05) centre (-10.439, -62.05) ccw projected
  circle A8 centre (-10.9, -45.3) radius 1.35 projected
  circle A9 centre (11.1, -45.3) radius 1.35 projected
  line L5 (-7.0991, -36.7384) -> (-5.1861, -28.9475) projected
  arc A10 (-2.575, -27.5395) -> (-5.1861, -28.9475) centre (-3.2438, -29.4244) ccw projected
  arc A11 (-2.575, -27.5395) -> (2.775, -27.5395) centre (0.1, -20) ccw projected
  arc A12 (5.3861, -28.9475) -> (2.775, -27.5395) centre (3.4438, -29.4244) ccw projected
  line L6 (5.3861, -28.9475) -> (7.2991, -36.7384) projected
  arc A13 (5.9409, -39.1281) -> (7.2991, -36.7384) centre (5.3568, -37.2153) ccw projected
  arc A14 (-5.7409, -39.1281) -> (5.9409, -39.1281) centre (0.1, -20) ccw projected
  arc A15 (-7.0991, -36.7384) -> (-5.7409, -39.1281) centre (-5.1568, -37.2153) ccw projected
  arc A16 (-3.802, -57.94) -> (-7.421, -58) centre (-5.611, -58) ccw projected
  line L7 (-3.802, -57.94) -> (4.08, -57.94) projected
  arc A17 (7.699, -58) -> (4.08, -57.94) centre (5.889, -58) ccw projected
  line L8 (7.699, -58) -> (7.699, -62) projected
  arc A18 (4.08, -62.06) -> (7.699, -62) centre (5.889, -62) ccw projected
  line L9 (4.08, -62.06) -> (-3.802, -62.06) projected
  arc A19 (-7.421, -62) -> (-3.802, -62.06) centre (-5.611, -62) ccw projected
  line L10 (-7.421, -62) -> (-7.421, -58) projected
  line L11 (8.16, -43.3) -> (8.16, -47.3) projected
  arc A20 (4.0409, -47.36) -> (8.16, -47.3) centre (6.1, -47.3) ccw projected
  line L12 (4.0409, -47.36) -> (-3.8409, -47.36) projected
  arc A21 (-7.96, -47.3) -> (-3.8409, -47.36) centre (-5.9, -47.3) ccw projected
  line L13 (-7.96, -47.3) -> (-7.96, -43.3) projected
  arc A22 (-3.8409, -43.24) -> (-7.96, -43.3) centre (-5.9, -43.3) ccw projected
  line L14 (-3.8409, -43.24) -> (4.0409, -43.24) projected
  arc A23 (8.16, -43.3) -> (4.0409, -43.24) centre (6.1, -43.3) ccw projected
  circle A24 centre (10.739, -60) radius 1.35 projected
  line L15 (-8.5217, -47.1327) -> (-4.4428, -30.5211) projected
  arc A25 (-0.2945, -27.4837) -> (-4.4428, -30.5211) centre (-0.5582, -31.475) ccw projected
  arc A26 (-0.2945, -27.4837) -> (0.6945, -27.4837) centre (0.2, -20) ccw projected
  arc A27 (4.8428, -30.5211) -> (0.6945, -27.4837) centre (0.9582, -31.475) ccw projected
  line L16 (4.8428, -30.5211) -> (8.9217, -47.1327) projected
  arc A28 (5.716, -52.0285) -> (8.9217, -47.1327) centre (5.0371, -48.0865) ccw projected
  arc A29 (-5.316, -52.0285) -> (5.716, -52.0285) centre (0.2, -20) ccw projected
  arc A30 (-8.5217, -47.1327) -> (-5.316, -52.0285) centre (-4.6371, -48.0865) ccw projected
  circle A31 centre (-10.261, -60) radius 1.35 projected
  line L17 (-7.261, -62) -> (-7.261, -58) projected
  arc A32 (-3.761, -58) -> (-7.261, -58) centre (-5.511, -58) ccw projected
  line L18 (-3.761, -58) -> (4.239, -58) projected
  arc A33 (7.739, -58) -> (4.239, -58) centre (5.989, -58) ccw projected
  line L19 (7.739, -58) -> (7.739, -62) projected
  arc A34 (4.239, -62) -> (7.739, -62) centre (5.989, -62) ccw projected
  line L20 (4.239, -62) -> (-3.761, -62) projected
  arc A35 (-7.261, -62) -> (-3.761, -62) centre (-5.511, -62) ccw projected
  circle A36 centre (0.2, -20) radius 4 projected
  arc A37 (-14.2236, -53.5801) -> (-14.339, -54.5339) centre (-10.339, -54.5339) ccw projected
  line L21 (-14.339, -54.5339) -> (-14.339, -62.05) projected
  arc A38 (-14.339, -62.05) -> (-10.339, -66.05) centre (-10.339, -62.05) ccw projected
  line L22 (-10.339, -66.05) -> (10.739, -66.05) projected
  arc A39 (10.739, -66.05) -> (14.739, -62.05) centre (10.739, -62.05) ccw projected
  line L23 (14.739, -62.05) -> (14.739, -54.5339) projected
  arc A40 (14.739, -54.5339) -> (14.6236, -53.5801) centre (10.739, -54.5339) ccw projected
  line L24 (14.6236, -53.5801) -> (6.0269, -18.5692) projected
  arc A41 (6.0269, -18.5692) -> (-5.6269, -18.5692) centre (0.2, -20) ccw projected
  line L25 (-5.6269, -18.5692) -> (-14.2236, -53.5801) projected
  line L26 (16.639, -62.05) -> (15.1111, -62.05)
  line L27 (15.1111, -62.05) -> (15.1111, -66.05)
  line L28 (15.1111, -66.05) -> (16.639, -66.05)
  line L29 (16.639, -66.05) -> (16.639, -62.05)
  line L30 (-14.9111, -66.05) -> (-16.439, -66.05)
  line L31 (-16.439, -66.05) -> (-16.439, -62.05)
  line L32 (-16.439, -62.05) -> (-14.9111, -62.05)
  line L33 (-14.9111, -62.05) -> (-14.9111, -66.05)
  point P0 (0, 0)
  constraints: 16 end point, 4 parallel, 2 perpendicular, 1 horizontal
extrude "돌출13" add sketch "스케치13" against normal up to surface (2 mm away) contours L30 L31 A7 | A3 L29 L28
fillet "모깎기6" radius 6 2 edges at (-16.439, -66.05, 1) (16.639, -66.05, 1)
sketch "스케치14" plane through (0, 0, 0) normal (0, 0, -1) x (-1, 0, 0)
  arc A0 (-16.639, -60.05) -> (-10.639, -66.05) centre (-10.639, -60.05) ccw projected
  line L0 (-10.639, -66.05) -> (10.439, -66.05) projected
  arc A1 (10.439, -66.05) -> (16.439, -60.05) centre (10.439, -60.05) ccw projected
  line L1 (16.439, -60.05) -> (16.439, -54.5339) projected
  arc A2 (16.439, -54.5339) -> (16.2659, -53.1031) centre (10.439, -54.5339) ccw projected
  line L2 (16.2659, -53.1031) -> (7.6692, -18.0923) projected
  arc A3 (7.6692, -18.0923) -> (-7.8692, -18.0923) centre (-0.1, -20) ccw projected
  line L3 (-7.8692, -18.0923) -> (-16.4659, -53.1031) projected
  arc A4 (-16.4659, -53.1031) -> (-16.639, -54.5339) centre (-10.639, -54.5339) ccw projected
  line L4 (-16.639, -54.5339) -> (-16.639, -60.05) projected
  line L5 (-8.16, -47.3) -> (-8.16, -43.3) projected
  arc A5 (-4.0409, -43.24) -> (-8.16, -43.3) centre (-6.1, -43.3) ccw projected
  line L6 (-4.0409, -43.24) -> (3.8409, -43.24) projected
  arc A6 (7.96, -43.3) -> (3.8409, -43.24) centre (5.9, -43.3) ccw projected
  line L7 (7.96, -43.3) -> (7.96, -47.3) projected
  arc A7 (3.8409, -47.36) -> (7.96, -47.3) centre (5.9, -47.3) ccw projected
  line L8 (3.8409, -47.36) -> (-4.0409, -47.36) projected
  arc A8 (-8.16, -47.3) -> (-4.0409, -47.36) centre (-6.1, -47.3) ccw projected
  arc A9 (7.421, -58) -> (3.802, -57.94) centre (5.611, -58) ccw projected
  line L9 (7.421, -58) -> (7.421, -62) projected
  arc A10 (3.802, -62.06) -> (7.421, -62) centre (5.611, -62) ccw projected
  line L10 (3.802, -62.06) -> (-4.08, -62.06) projected
  arc A11 (-7.699, -62) -> (-4.08, -62.06) centre (-5.889, -62) ccw projected
  line L11 (-7.699, -62) -> (-7.699, -58) projected
  arc A12 (-4.08, -57.94) -> (-7.699, -58) centre (-5.889, -58) ccw projected
  line L12 (-4.08, -57.94) -> (3.802, -57.94) projected
  line L13 (5.1861, -28.9475) -> (7.0991, -36.7384) projected
  arc A13 (5.7409, -39.1281) -> (7.0991, -36.7384) centre (5.1568, -37.2153) ccw projected
  arc A14 (-5.9409, -39.1281) -> (5.7409, -39.1281) centre (-0.1, -20) ccw projected
  arc A15 (-7.2991, -36.7384) -> (-5.9409, -39.1281) centre (-5.3568, -37.2153) ccw projected
  line L14 (-7.2991, -36.7384) -> (-5.3861, -28.9475) projected
  arc A16 (-2.775, -27.5395) -> (-5.3861, -28.9475) centre (-3.4438, -29.4244) ccw projected
  arc A17 (-2.775, -27.5395) -> (2.575, -27.5395) centre (-0.1, -20) ccw projected
  arc A18 (5.1861, -28.9475) -> (2.575, -27.5395) centre (3.2438, -29.4244) ccw projected
  circle A19 centre (-11.1, -45.3) radius 1.35 projected
  circle A20 centre (10.9, -45.3) radius 1.35 projected
  circle A21 centre (-0.1, -20) radius 4 projected
  circle A22 centre (-10.639, -60) radius 1.35 projected
  circle A23 centre (10.361, -60) radius 1.35 projected
  point P0 (0, 0)
extrude "돌출14" add sketch "스케치14" against normal up to surface (2 mm away) contours L9 A10 L10 A11 L11 A12 L12 A9
sketch "스케치15" plane through (0, 0, 0) normal (0, 0, -1) x (-1, 0, 0)
  line L0 (6.921, -57.5) -> (6.921, -59.5) projected
  arc A0 (4.7026, -59.56) -> (6.921, -59.5) centre (5.811, -59.5) ccw projected
  line L1 (4.7026, -59.56) -> (-3.9306, -59.56) projected
  arc A1 (-6.149, -59.5) -> (-3.9306, -59.56) centre (-5.039, -59.5) ccw projected
  line L2 (-6.149, -59.5) -> (-6.149, -57.5) projected
  arc A2 (-3.9306, -57.44) -> (-6.149, -57.5) centre (-5.039, -57.5) ccw projected
  line L3 (-3.9306, -57.44) -> (4.7026, -57.44) projected
  arc A3 (6.921, -57.5) -> (4.7026, -57.44) centre (5.811, -57.5) ccw projected
  line L4 (-14.6916, -62.5) -> (14.3356, -62.5) projected
  arc A4 (14.3356, -62.5) -> (14.361, -62.05) centre (10.361, -62.05) ccw projected
  line L5 (14.361, -62.05) -> (14.361, -54.5339) projected
  arc A5 (14.361, -54.5339) -> (14.2456, -53.5801) centre (10.361, -54.5339) ccw projected
  line L6 (14.2456, -53.5801) -> (5.6489, -18.5692) projected
  arc A6 (5.6489, -18.5692) -> (-6.0049, -18.5692) centre (-0.178, -20) ccw projected
  line L7 (-6.0049, -18.5692) -> (-14.6016, -53.5801) projected
  arc A7 (-14.6016, -53.5801) -> (-14.717, -54.5339) centre (-10.717, -54.5339) ccw projected
  line L8 (-14.717, -54.5339) -> (-14.717, -62.05) projected
  arc A8 (-14.717, -62.05) -> (-14.6916, -62.5) centre (-10.717, -62.05) ccw projected
  circle A9 centre (10.361, -60) radius 1.35 projected
  line L9 (-8.8997, -47.1327) -> (-4.8208, -30.5211) projected
  arc A10 (-0.6725, -27.4837) -> (-4.8208, -30.5211) centre (-0.9362, -31.475) ccw projected
  arc A11 (-0.6725, -27.4837) -> (0.3165, -27.4837) centre (-0.178, -20) ccw projected
  arc A12 (4.4648, -30.5211) -> (0.3165, -27.4837) centre (0.5802, -31.475) ccw projected
  line L10 (4.4648, -30.5211) -> (8.5437, -47.1327) projected
  arc A13 (5.3379, -52.0285) -> (8.5437, -47.1327) centre (4.6591, -48.0865) ccw projected
  arc A14 (-5.694, -52.0285) -> (5.3379, -52.0285) centre (-0.178, -20) ccw projected
  arc A15 (-8.8997, -47.1327) -> (-5.694, -52.0285) centre (-5.0151, -48.0865) ccw projected
  circle A16 centre (-10.639, -60) radius 1.35 projected
  circle A17 centre (-0.178, -20) radius 4 projected
  arc A18 (-16.639, -60.05) -> (-10.639, -66.05) centre (-10.639, -60.05) ccw projected
  line L11 (-10.639, -66.05) -> (10.439, -66.05) projected
  arc A19 (10.439, -66.05) -> (16.439, -60.05) centre (10.439, -60.05) ccw projected
  line L12 (16.439, -60.05) -> (16.439, -54.5339) projected
  arc A20 (16.439, -54.5339) -> (16.2659, -53.1031) centre (10.439, -54.5339) ccw projected
  line L13 (16.2659, -53.1031) -> (7.6692, -18.0923) projected
  arc A21 (7.6692, -18.0923) -> (-7.8692, -18.0923) centre (-0.1, -20) ccw projected
  line L14 (-7.8692, -18.0923) -> (-16.4659, -53.1031) projected
  arc A22 (-16.4659, -53.1031) -> (-16.639, -54.5339) centre (-10.639, -54.5339) ccw projected
  line L15 (-16.639, -54.5339) -> (-16.639, -60.05) projected
  line L16 (-8.16, -47.3) -> (-8.16, -43.3) projected
  arc A23 (-4.0409, -43.24) -> (-8.16, -43.3) centre (-6.1, -43.3) ccw projected
  line L17 (-4.0409, -43.24) -> (3.8409, -43.24) projected
  arc A24 (7.96, -43.3) -> (3.8409, -43.24) centre (5.9, -43.3) ccw projected
  line L18 (7.96, -43.3) -> (7.96, -47.3) projected
  arc A25 (3.8409, -47.36) -> (7.96, -47.3) centre (5.9, -47.3) ccw projected
  line L19 (3.8409, -47.36) -> (-4.0409, -47.36) projected
  arc A26 (-8.16, -47.3) -> (-4.0409, -47.36) centre (-6.1, -47.3) ccw projected
  line L20 (5.1861, -28.9475) -> (7.0991, -36.7384) projected
  arc A27 (5.7409, -39.1281) -> (7.0991, -36.7384) centre (5.1568, -37.2153) ccw projected
  arc A28 (-5.9409, -39.1281) -> (5.7409, -39.1281) centre (-0.1, -20) ccw projected
  arc A29 (-7.2991, -36.7384) -> (-5.9409, -39.1281) centre (-5.3568, -37.2153) ccw projected
  line L21 (-7.2991, -36.7384) -> (-5.3861, -28.9475) projected
  arc A30 (-2.775, -27.5395) -> (-5.3861, -28.9475) centre (-3.4438, -29.4244) ccw projected
  arc A31 (-2.775, -27.5395) -> (2.575, -27.5395) centre (-0.1, -20) ccw projected
  arc A32 (5.1861, -28.9475) -> (2.575, -27.5395) centre (3.2438, -29.4244) ccw projected
  circle A33 centre (-11.1, -45.3) radius 1.35 projected
  circle A34 centre (10.9, -45.3) radius 1.35 projected
  circle A35 centre (-0.1, -20) radius 4 projected
  circle A36 centre (-10.639, -60) radius 1.35 projected
  circle A37 centre (10.361, -60) radius 1.35 projected
  line L22 (-14.6916, -62.5) -> (-22.0036, -62.5)
  line L23 (-14.6916, -62.5) -> (-7.3797, -62.5) construction
  line L24 (-22.0036, -62.5) -> (27.0848, -62.5)
  point P0 (0, 0)
  point P1 (15.916, -62.5)
  point P2 (-16.116, -62.5)
  dimension "d59" = 180
  constraints: 6 end point, 1 collinear, 1 horizontal, 1 point on line
  measures "d59" angle of L22 L23
extrude "돌출15" cut sketch "스케치15" against normal through all contours L0 A0 L1 A1 L2 A2 L3 A3 | L4 L24 A19 L11 A18 L22